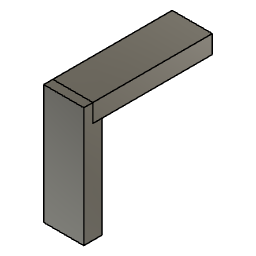
Rebate Joint (Autodesk Fusion 360 design; units mm, degrees)
Autodesk Fusion 360 part; units mm, degrees
sketch "First piece" plane through (0, 0, 0) normal (0, 1, 0) x (1, 0, 0)
  line L0 (0, 0) -> (-42, 0)
  line L1 (-42, 0) -> (-42, -125)
  line L2 (-42, -125) -> (0, -125)
  line L3 (0, -125) -> (0, 0)
  dimension "d6" = 42
  dimension "d7" = 125
  constraint horizontal L0
  constraint vertical L1
  constraint horizontal L2
  constraint vertical L3
  constraint coincident L0.start L3.end
  measures "d6" distance of L0.start L0.end
  measures "d7" distance of L0.start L2.end
extrude "Extrude1" add sketch "First piece" along normal blind 19 makes body 1
sketch "Cut" plane through (0, 19, 0) normal (0, 1, 0) x (-1, 0, 0)
  line L0 (0, 125) -> (0, 0)
  line L1 (0, 0) -> (42, 0)
  line L2 (42, 0) -> (42, 125)
  line L3 (42, 125) -> (0, 125)
  line L4 (42, 125) -> (0, 125)
  line L5 (0, 125) -> (0, 106)
  line L6 (0, 106) -> (42, 106)
  line L7 (42, 106) -> (42, 125)
  dimension "d10" = 42
  dimension "d11" = 19
  constraint horizontal L4
  constraint vertical L5
  constraint horizontal L6
  constraint vertical L7
  constraint coincident L2.end L3.start
  measures "d10" distance of L2.end L0.start
  measures "d11" distance of L2.end L6.end
extrude "Extrude2" cut sketch "Cut" against normal blind 9.5 contours L0 L2 L3 L4 L5 L6 L7 bodies 1
copy_body "Body->Comp1" bodies 1 removing the originals makes body 2 in component "First Piece"
sketch "Second Piece" plane through (0, 9.5, 0) normal (0, 1, 0) x (-1, 0, 0)
  line L0 (42, 106) -> (42, 125)
  line L1 (42, 125) -> (0, 125)
  line L2 (0, 125) -> (0, 106)
  line L3 (0, 106) -> (42, 106)
  line L4 (0, 125) -> (42, 125)
  line L5 (42, 125) -> (42, 106)
  line L6 (42, 106) -> (0, 106)
  line L7 (0, 106) -> (0, 125)
  constraint horizontal L4
  constraint vertical L5
  constraint horizontal L6
  constraint vertical L7
  constraint coincident L0.start L3.end
  constraint coincident L1.end L2.start
extrude "Extrude1'" add sketch "Second Piece" along normal blind 125 separate body makes body 3 in component "Second Piece"
component "First Piece" placed x (1, 0, 0) y (0, 1, 0) z (0, 0, 1) at (0, 0, 0)
component "Second Piece" placed x (1, 0, 0) y (0, 1, 0) z (0, 0, 1) at (0, 0, 0)
equation "lenght = 125 mm"
equation "width = 42 mm"
equation "thickness = 19 mm"
equation "d6 = width"
equation "d7 = lenght"
equation "d8 = thickness"
equation "d10 = width"
equation "d11 = thickness"
equation "d12 = -thickness / 2"
equation "d14 = lenght"
named bodies: "First Piece", "Second Piece"
